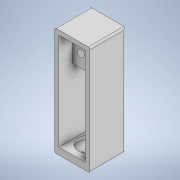
# Autodesk Inventor part: Link5_v2
Saved by Autodesk Inventor 2022 (Build 260153000, 153)
## iProperties
Created: 2022-06-14
Part Number: Link5_v2
Material: Generic
Document SubType Name: Modeling
Designer: Asus
Density: 1 g/cm^3
Appearance: Default
Author: Asus
Autodesk Inventor part; units mm, degrees
ref_plane "YZ Plane" through (0, 0, 0) normal (1, 0, 0) x (0, 1, 0)
ref_plane "XZ Plane" through (0, 0, 0) normal (0, 1, 0) x (-1, 0, 0)
ref_plane "XY Plane" through (0, 0, 0) normal (0, 0, 1) x (1, 0, 0)
sketch "Sketch1" plane through (0, 0, 0) normal (0, 0, 1) x (1, 0, 0)
  line L0 (-20, 22.5) -> (20, 22.5)
  line L1 (20, 22.5) -> (20, -100)
  line L2 (20, -100) -> (-20, -100)
  line L3 (-20, -100) -> (-20, 22.5)
  circle A0 centre (0, 0) radius 4
  dimension "d0" = 122.5
  dimension "d1" = 40
  dimension "d2" = 20
  dimension "d3" = 22.5
  dimension "d4" = 8
  constraints: 8 end point, 2 parallel, 1 centre point, 1 coincident, 1 horizontal, 1 perpendicular
  measures "d0" distance of L0.end L1.end
  measures "d1" distance of L0.start L0.end
  measures "d2" distance from line of point (0, 0) L1
  measures "d3" distance from line of L0 point (0, 0)
  measures "d4" diameter of A0
extrude "Extrusion1" add sketch "Sketch1" along normal blind 5
sketch "Sketch2" plane through (0, 0, 5) normal (0, 0, 1) x (1, 0, 0)
  line L0 (20, 22.5) -> (-20, 22.5) projected
  line L1 (-20, -100) -> (20, -100) projected
  line L2 (-20, 22.5) -> (20, 22.5)
  line L3 (20, 22.5) -> (20, -100)
  line L4 (20, -100) -> (-20, -100)
  line L5 (-20, -100) -> (-20, 22.5)
  line L6 (-15, 17.5) -> (15, 17.5)
  line L7 (15, 17.5) -> (15, -95)
  line L8 (15, -95) -> (-15, -95)
  line L9 (-15, -95) -> (-15, 17.5)
  point P0 (0, 0)
  dimension "d7" = 5
  dimension "d8" = 5
  dimension "d9" = 5
  dimension "d10" = 5
  constraints: 16 end point, 4 parallel, 2 horizontal, 2 perpendicular
  measures "d7" distance between parallel lines of L3 L7
  measures "d8" distance between parallel lines of L5 L9
  measures "d9" distance between parallel lines of L8 L1
  measures "d10" distance between parallel lines of L0 L6
extrude "Extrusion2" add sketch "Sketch2" along normal blind 35
sketch "Sketch3" plane through (-20, -100, 0) normal (0, -1, 0) x (1, 0, 0)
  circle A0 centre (20, 20) radius 4
  line L0 (40, 0) -> (40, 40) projected
  line L1 (0, 0) -> (40, 0) projected
  circle A1 centre (20, 20) radius 8.5
  line L2 (9.176, 20) -> (31.9076, 20)
  circle A2 centre (11.5, 20) radius 1.5
  circle A3 centre (28.5, 20) radius 1.5
  line L3 (0, 40) -> (40, 40) projected
  line L4 (20, 9.4564) -> (20, 30.2603)
  circle A4 centre (20, 28.5) radius 1.5
  circle A5 centre (20, 11.5) radius 1.5
  point P0 (20, 0)
  dimension "d13" = 20
  dimension "d14" = 20
  dimension "d15" = 8
  dimension "d16" = 17
  dimension "d17" = 3
  dimension "d18" = 3
  dimension "d19" = 20
  dimension "d20" = 20
  dimension "d21" = 3
  dimension "d22" = 3
  constraints: 6 centre point, 4 end point, 4 point on circle, 4 point on line, 1 coincident, 1 horizontal, 1 vertical
  measures "d13" distance from line of L0 A0.centre
  measures "d14" distance from line of L1 A0.centre
  measures "d15" diameter of A0
  measures "d16" diameter of A1
  measures "d17" diameter of A3
  measures "d18" diameter of A2
  measures "d19" distance from line of L3 A2.centre
  measures "d20" distance between parallel lines of L0 L4
  measures "d21" diameter of A5
  measures "d22" diameter of A4
extrude "Extrusion3" cut sketch "Sketch3" against normal blind 10 contours L2 L4 A0 | A0 L4 L2 | L4 L2 A0 | A0 L2 L4 | A4 A1 L4 | L4 A1 A4 | A5 A1 L4 | L4 A1 A5 | L4 A4 A1 | A1 A4 L4 | L4 A5 A1 | A1 A5 L4
sketch "Sketch4" plane through (-15, -95, 5) normal (0, 1, 0) x (1, 0, 0)
  line L0 (0, 0) -> (30, 0)
  line L1 (30, 0) -> (30, -35)
  line L2 (30, -35) -> (0, -35)
  line L3 (0, -35) -> (0, 0)
  circle A0 centre (15, -15) radius 4 projected
  circle A1 centre (15, -15) radius 13
  circle A2 centre (15, -23.5) radius 1.5 projected
  circle A3 centre (15, -23.5) radius 1.5
  circle A4 centre (15, -6.5) radius 1.5 projected
  circle A5 centre (15, -6.5) radius 1.5
  point P0 (15, 5)
  dimension "d25" = 26
  constraints: 8 end point, 3 centre point, 3 coincident, 2 parallel, 1 horizontal, 1 perpendicular
  measures "d25" diameter of A1
extrude "Extrusion4" add sketch "Sketch4" along normal blind 3 contours L0 L1 L2 L3 | A1
sketch "Sketch5" plane through (-15, -92, 5) normal (0, 1, 0) x (1, 0, 0)
  circle A0 centre (15, -15) radius 4 projected
  circle A1 centre (15, -15) radius 13
  point P0 (15, 5)
  dimension "d28" = 26
  constraints: 1 centre point, 1 coincident
  measures "d28" diameter of A1
extrude "Extrusion5" cut sketch "Sketch5" against normal blind 4
fillet "Fillet1" radius 2 5 edges at (-20, 22.5, 20) (20, 22.5, 20) (20, -100, 20) (-20, -100, 20) (20, -38.75, 0)
sketch "Sketch6" plane through (0, 0, 5) normal (0, 0, 1) x (1, 0, 0)
  line L0 (-15, -92) -> (-15, 17.5) projected
  line L1 (15, 17.5) -> (15, -92) projected
  line L2 (-15, 17.5) -> (15, 17.5)
  line L3 (15, 17.5) -> (15, -17.5)
  line L4 (15, -17.5) -> (-15, -17.5)
  line L5 (-15, -17.5) -> (-15, 17.5)
  circle A0 centre (0, 0) radius 4
  point P0 (-15, -17.5)
  dimension "d32" = 35
  constraints: 8 end point, 2 parallel, 1 centre point, 1 coincident, 1 horizontal, 1 perpendicular, 1 point on line
  measures "d32" distance between parallel lines of L2 L4
extrude "Extrusion6" add sketch "Sketch6" along normal blind 20
sketch "Sketch7" plane through (0, 0, 0) normal (0, 0, -1) x (-1, 0, 0)
  circle A0 centre (0, 0) radius 9.5
  dimension "d35" = 19
  constraints: 1 centre point, 1 coincident
  measures "d35" diameter of A0
extrude "Extrusion7" cut sketch "Sketch7" against normal blind 12.5
sketch "Sketch8" plane through (0, 0, 0) normal (0, 0, -1) x (-1, 0, 0)
  circle A0 centre (0, 0) radius 4 projected
  circle A1 centre (0, 0) radius 11.5
  dimension "d38" = 23
  constraints: 1 centre point, 1 coincident
  measures "d38" diameter of A1
extrude "Extrusion8" cut sketch "Sketch8" against normal blind 6.5
sketch "Sketch9" plane through (0, 0, 25) normal (0, 0, 1) x (1, 0, 0)
  circle A0 centre (0, 0) radius 4
  constraints: 1 centre point, 1 coincident
extrude "Extrusion9" add sketch "Sketch9" against normal blind 12.5
sketch "Sketch10" plane through (0, 0, 12.5) normal (0, 0, -1) x (-1, 0, 0)
  circle A0 centre (0, 0) radius 6.2
  line L0 (0, 6.2) -> (0, 0)
  line L1 (0, 0) -> (6.261, -3.6148)
  line L2 (0, 0) -> (-6.878, -3.971)
  circle A1 centre (0, 6.2) radius 1.45
  circle A2 centre (5.3694, -3.1) radius 1.45
  circle A3 centre (-5.3694, -3.1) radius 1.45
  dimension "d43" = 12.4
  dimension "d44" = 120
  dimension "d45" = 120
  dimension "d46" = 2.9
  dimension "d47" = 2.9
  dimension "d48" = 2.9
  constraints: 6 end point, 4 centre point, 3 point on circle, 2 coincident, 2 point on line, 1 vertical
  measures "d43" diameter of A0
  measures "d44" angle of L0 L2
  measures "d45" angle of L1 L2
  measures "d46" diameter of A1
  measures "d47" diameter of A2
  measures "d48" diameter of A3
extrude "Extrusion10" cut sketch "Sketch10" against normal blind 12.5 contours A1 L0 A0 | A0 A1 | A2 A0 | A0 L1 A2 | L0 A1 A0 | A0 A2 L1 | A3 L2 A0 | A0 L2 A3 | A3 A0 L2 | A3 L2 A0
sketch "Sketch11" plane through (0, 0, 25) normal (0, 0, 1) x (1, 0, 0)
  circle A0 centre (5.3694, -3.1) radius 1.45 projected
  circle A1 centre (5.3694, -3.1) radius 4
  circle A2 centre (-5.3694, -3.1) radius 1.45 projected
  circle A3 centre (-5.3694, -3.1) radius 4
  circle A4 centre (0, 6.2) radius 1.45 projected
  circle A5 centre (0, 6.2) radius 4
  point P0 (0, 0)
  dimension "d51" = 8
  dimension "d52" = 8
  dimension "d53" = 8
  constraints: 3 centre point, 3 coincident
  measures "d51" diameter of A5
  measures "d52" diameter of A1
  measures "d53" diameter of A3
extrude "Extrusion11" cut sketch "Sketch11" against normal blind 7
body "Solid1"
